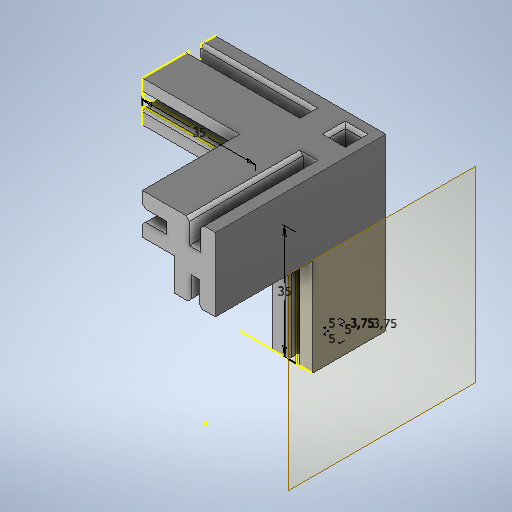
# Autodesk Inventor part: Kątownk Środek LEWY Plexa
Saved by Autodesk Inventor 2025 (Build 290162000, 162)
## iProperties
Created: 2025-07-29
Part Number: Kątownk Środek LEWY Plexa
Material: Ogólny
Document SubType Name: Modeling
Designer: ThePi
Density: 1 g/cm^3
Appearance: Domyślna
Author: ThePi
Autodesk Inventor part; units mm, degrees
(part 1 of 2)
ref_plane "YZ Plane" through (0, 0, 0) normal (1, 0, 0) x (0, 1, 0)
ref_plane "XZ Plane" through (0, 0, 0) normal (0, 1, 0) x (-1, 0, 0)
ref_plane "XY Plane" through (0, 0, 0) normal (0, 0, 1) x (1, 0, 0)
sketch "Szkic1" plane through (0, 0, 0) normal (0, 1, 0) x (-1, 0, 0)
  line L0 (0, 0) -> (0, 15)
  line L1 (0, 15) -> (0, 0)
  line L2 (0, 0) -> (15, 0)
  line L3 (3, 10) -> (4.25, 10)
  line L4 (3, 10) -> (1.75, 10)
  line L5 (1.75, 10) -> (1.75, 15)
  line L6 (4.25, 10) -> (4.25, 15)
  line L7 (1.75, 15) -> (-3.25, 15)
  line L8 (4.25, 15) -> (9.25, 15)
  line L9 (-3.25, 15) -> (-3.25, 0)
  line L10 (-3.25, 0) -> (15, 0)
  line L11 (-3.25, 0) -> (11.75, 0)
  line L12 (9.25, 15) -> (9.25, 5)
  line L13 (9.25, 5) -> (19.25, 5)
  line L14 (19.25, 5) -> (19.25, 0)
  line L15 (19.25, 0) -> (14.25, 0)
  line L16 (14.25, 0) -> (14.25, -2.5)
  line L17 (14.25, -2.5) -> (19.25, -2.5)
  line L18 (19.25, -2.5) -> (19.25, -7.5)
  line L19 (19.25, -7.5) -> (9.25, -7.5)
  line L20 (-3.25, 0) -> (-3.25, -7.5)
  line L21 (-3.25, -7.5) -> (9.25, -7.5)
  line L22 (3, 10) -> (3, -1.25)
  line L23 (3, -1.25) -> (14.25, -1.25)
  dimension "d0" = 15
  dimension "d6" = 1.25
  dimension "d7" = 1.25
  dimension "d9" = 5
  dimension "d10" = 5
  dimension "d13" = 10
  dimension "d14" = 10
  dimension "d15" = 5
  dimension "d16" = 5
  dimension "d17" = 2.5
  dimension "d18" = 5
  dimension "d19" = 10
  constraints: 48 end point, 7 perpendicular, 5 point on line, 4 vertical, 2 collinear, 2 horizontal, 1 midpoint, 1 parallel
  measures "d0" distance of L0.start L0.end
  measures "d6" distance of L3.start L3.end
  measures "d7" distance of L3.start L4.end
  measures "d9" distance of L5.end L7.end
  measures "d10" distance of L6.end L8.end
  measures "d13" distance of L8.end L12.end
  measures "d14" distance of L12.end L13.end
  measures "d15" distance of L13.end L14.end
  measures "d16" distance of L14.end L15.end
  measures "d17" distance of L15.end L16.end
  measures "d18" distance of L17.end L18.end
  measures "d19" distance of L18.end L19.end
extrude "Wyciągnięcie proste1" add sketch "Szkic1" along normal blind 30
sketch "Szkic2" plane through (0, 30, 0) normal (0, 1, 0) x (1, 0, 0)
  line L0 (3.25, 7.5) -> (-19.25, 7.5) projected
  line L1 (-19.25, -5) -> (-9.25, -5) projected
  line L2 (-19.25, 7.5) -> (-19.25, -5)
  line L3 (-19.25, -5) -> (-9.25, -5)
  line L4 (-9.25, -5) -> (-9.25, -15) projected
  line L5 (-9.25, -5) -> (-9.25, -15)
  line L6 (-1.75, -15) -> (3.25, -15) projected
  line L7 (-9.25, -15) -> (3.25, -15)
  line L8 (3.25, -15) -> (3.25, 7.5)
  line L9 (3.25, 7.5) -> (-19.25, 7.5)
  point P0 (0, 0)
  constraints: 12 end point, 3 perpendicular, 2 collinear, 1 vertical
extrude "Wyciągnięcie proste2" add sketch "Szkic2" along normal blind 30
sketch "Szkic3" plane through (0, 0, 0) normal (0, -1, 0) x (1, 0, 0)
  point P0 (0, 0)
sketch "Szkic4" plane through (-19.25, 0, -7.5) normal (-1, 0, 0) x (0, 0, 1)
  line L0 (0, 30) -> (12.5, 30)
  line L1 (12.5, 0) -> (12.5, 60) projected
  line L2 (12.5, 30) -> (12.5, 60)
  line L3 (12.5, 60) -> (0, 60)
  line L4 (0, 60) -> (0, 30)
  point P0 (7.5, 0)
  constraints: 8 end point, 2 perpendicular, 1 collinear, 1 midpoint
extrude "Wyciągnięcie proste3" add sketch "Szkic4" along normal blind 30
sketch "Szkic5" plane through (-9.25, 0, 5) normal (-1, 0, 0) x (0, 0, 1)
  line L0 (10, 0) -> (10, 60) projected
  line L1 (10, 30) -> (5, 30) projected
  line L2 (10, 60) -> (10, 30)
  line L3 (10, 30) -> (0, 30)
  line L4 (0, 30) -> (0, 60)
  line L5 (0, 60) -> (10, 60)
  point P0 (-5, 0)
  constraints: 8 end point, 2 perpendicular, 1 collinear, 1 vertical
extrude "Wyciągnięcie proste4" add sketch "Szkic5" along normal up to surface (40 mm away)
sketch "Szkic6" plane through (0, 30, 0) normal (0, -1, 0) x (1, 0, 0)
  line L0 (-14.25, 0) -> (-19.25, 0) projected
  line L1 (-14.25, 0) -> (-49.25, 0)
  line L2 (-49.25, -7.5) -> (-49.25, 15) projected
  line L3 (-49.25, 0) -> (-49.25, -2.5)
  line L4 (-49.25, -2.5) -> (-14.25, -2.5)
  line L5 (-14.25, -2.5) -> (-14.25, 0)
  line L6 (-14.25, 10) -> (-49.25, 10)
  line L7 (-4.25, 10) -> (-1.75, 10) projected
  point P0 (0, 0)
  constraints: 10 end point, 3 point on line, 2 perpendicular, 1 collinear, 1 horizontal, 1 vertical
extrude "Wyciągnięcie proste5" cut sketch "Szkic6" against normal blind 5
sketch "Szkic7" plane through (-1.75, 0, 15) normal (0, 0, 1) x (1, 0, 0)
  line L0 (-7.5, 30) -> (-17.5, 30) projected
  line L1 (-7.5, 30) -> (-17.5, 30)
  line L2 (-7.5, 30) -> (-7.5, 40)
  line L3 (5, 0) -> (5, 60) projected
  line L4 (-7.5, 30) -> (2.5, 30) construction
  line L5 (-7.5, 40) -> (-47.5, 40)
  line L6 (-47.5, 60) -> (-47.5, 30) projected
  line L7 (-47.5, 40) -> (-47.5, 30)
  line L8 (-47.5, 30) -> (-7.5, 30)
  point P0 (1.75, 0)
  dimension "d30" = 10
  dimension "d31" = 10
  dimension "d32" = 90
  constraints: 12 end point, 2 collinear, 2 perpendicular, 1 horizontal, 1 parallel, 1 point on line, 1 vertical
  measures "d30" distance of L0.start L0.end
  measures "d31" distance of L0.start L2.end
  measures "d32" angle of L4 L2
extrude "Wyciągnięcie proste6" cut sketch "Szkic7" against normal up to surface (10 mm away)
sketch "Szkic8" plane through (-49.25, 0, -7.5) normal (-1, 0, 0) x (0, 0, 1)
  point P0 (7.5, 0)
sketch "Szkic9" plane through (0, 0, 0) normal (0, -1, 0) x (1, 0, 0)
  point P0 (0, 0)
sketch "Szkic10" plane through (-49.25, 0, -7.5) normal (-1, 0, 0) x (0, 0, 1)
  line L0 (0, 0) -> (0, 60) projected
  line L1 (0, 30) -> (0, 52.5)
  line L2 (0, 52.5) -> (22.5, 52.5)
  line L3 (22.5, 0) -> (22.5, 60) projected
  line L4 (22.5, 52.5) -> (22.5, 40)
  line L5 (22.5, 40) -> (12.5, 40)
  line L6 (12.5, 40) -> (12.5, 30)
  line L7 (0, 30) -> (5, 30) projected
  line L8 (12.5, 30) -> (0, 30)
  line L9 (22.5, 52.5) -> (22.5, 60)
  line L10 (22.5, 60) -> (0, 60) projected
  line L11 (0, 60) -> (0, 52.5)
  line L12 (22.5, 52.5) -> (0, 52.5)
  point P0 (7.5, 0)
  dimension "d35" = 22.5
  dimension "d36" = 90
  dimension "d37" = 10
  constraints: 18 end point, 4 perpendicular, 3 collinear, 2 point on line, 1 midpoint
  measures "d35" distance of L1.start L1.end
  measures "d36" angle of L1 L2
  measures "d37" distance of L4.end L5.end
sketch "Szkic11" plane through (0, 0, 0) normal (0, -1, 0) x (1, 0, 0)
  point P0 (0, 0)
extrude "Wyciągnięcie proste7" cut sketch "Szkic10" against normal up to surface (52.5 mm away) contours L0 L10 L3 L2
sketch "Szkic12" plane through (-9.25, 0, 15) normal (0, 0, 1) x (1, 0, 0)
  line L0 (12.5, 52.5) -> (-40, 52.5) projected
  line L1 (12.5, 52.5) -> (-10, 52.5)
  line L2 (-10, 30) -> (-40, 30) projected
  line L3 (-10, 52.5) -> (-10, 30)
  line L4 (-10, 30) -> (12.5, 30)
  line L5 (12.5, 0) -> (12.5, 52.5) projected
  line L6 (12.5, 30) -> (12.5, 52.5)
  line L7 (-10, 30) -> (-10, 40)
  line L8 (-40, 40) -> (0, 40) projected
  line L9 (0, 40) -> (0, 30.3734)
  line L10 (0, 0) -> (0, 40) projected
  point P0 (9.25, 0)
  point P1 (0, 30)
  point P2 (0, 40)
  constraints: 12 end point, 3 perpendicular, 3 point on line, 1 parallel
extrude "Wyciągnięcie proste8" add sketch "Szkic12" against normal blind 10 contours L8 L9 L10 L4 L3
sketch "Szkic13" plane through (-9.25, 0, 15) normal (0, 0, 1) x (1, 0, 0)
  line L0 (-40, 52.5) -> (-40, 40) projected
  line L1 (-40, 40) -> (-40, 45)
  line L2 (-40, 45) -> (-10, 45)
  line L3 (-10, 45) -> (-10, 47.5)
  line L4 (-10, 47.5) -> (-40, 47.5)
  line L5 (12.5, 52.5) -> (-40, 52.5) projected
  line L6 (-40, 52.5) -> (-40, 47.5)
  line L7 (-40, 45) -> (-40, 47.5)
  point P0 (9.25, 0)
  dimension "d42" = 5
  dimension "d43" = 30
  dimension "d44" = 2.5
  constraints: 12 end point, 2 collinear, 2 perpendicular, 2 point on line, 1 horizontal
  measures "d42" distance of L0.end L1.end
  measures "d43" distance of L1.end L2.end
  measures "d44" distance of L2.end L3.end
extrude "Wyciągnięcie proste9" cut sketch "Szkic13" against normal blind 5
sketch "Szkic14" plane through (-9.25, 0, 15) normal (0, 0, 1) x (1, 0, 0)
  line L0 (12.5, 0) -> (12.5, 52.5) projected
  line L1 (12.5, 52.5) -> (-10, 52.5)
  line L2 (12.5, 52.5) -> (-40, 52.5) projected
  line L3 (-10, 40) -> (-10, 30) projected
  line L4 (-10, 52.5) -> (-10, 30)
  line L5 (-10, 30) -> (12.5, 30)
  line L6 (12.5, 30) -> (12.5, 52.5)
  point P0 (9.25, 0)
  constraints: 8 end point, 2 perpendicular, 1 point on line, 1 vertical
extrude "Wyciągnięcie proste10" add sketch "Szkic14" along normal blind 30
sketch "Szkic15" plane through (-1.75, 0, 15) normal (0, 0, 1) x (1, 0, 0)
  line L0 (0, 0) -> (0, 30) projected
  line L1 (0, 0) -> (0, 35)
  line L2 (0, 35) -> (0, 0)
  line L3 (-2.5, 0) -> (-2.5, 30) projected
  line L4 (0, 0) -> (-2.5, 0)
  line L5 (5, 0) -> (-17.5, 0) projected
  line L6 (-2.5, 0) -> (-2.5, 35)
  line L7 (-2.5, 35) -> (0, 35)
  line L8 (0, 0) -> (0, 35)
  line L9 (-17.5, 45) -> (-47.5, 45) projected
  line L10 (-47.5, 45) -> (-12.5, 45)
  line L11 (-12.5, 45) -> (-47.5, 45)
  line L12 (-47.5, 47.5) -> (-17.5, 47.5) projected
  line L13 (-47.5, 45) -> (-47.5, 47.5)
  line L14 (-47.5, 47.5) -> (-12.5, 47.5)
  line L15 (-12.5, 47.5) -> (-12.5, 45)
  point P0 (1.75, 0)
  point P1 (-17.5, 47.5)
  dimension "d49" = 35
  dimension "d50" = 35
  constraints: 22 end point, 6 collinear, 2 perpendicular, 2 vertical, 1 parallel
  measures "d49" distance of L0.start L1.end
  measures "d50" distance of L9.end L10.end
extrude "Wyciągnięcie proste11" cut sketch "Szkic15" against normal up to surface (5 mm away)
sketch "Szkic16" plane through (-9.25, 0, 45) normal (0, 0, 1) x (1, 0, 0)
  line L0 (7.5, 0) -> (7.5, 35) projected
  line L1 (7.5, 30) -> (7.5, 35)
  line L2 (5, 35) -> (5, 30) projected
  line L3 (7.5, 35) -> (5, 35)
  line L4 (5, 35) -> (5, 30)
  line L5 (5, 30) -> (7.5, 30)
  line L6 (-10, 40) -> (-10, 45) projected
  line L7 (-10, 45) -> (-5, 45) projected
  line L8 (-10, 45) -> (-5, 45)
  line L9 (-5, 47.5) -> (-10, 47.5) projected
  line L10 (-5, 45) -> (-5, 47.5)
  line L11 (-5, 47.5) -> (-10, 47.5)
  line L12 (-10, 47.5) -> (-10, 45)
  point P0 (9.25, 0)
  dimension "d53" = 5
  constraints: 16 end point, 5 perpendicular, 3 collinear, 1 point on line
  measures "d53" distance of L1.start L0.end
extrude "Wyciągnięcie proste12" cut sketch "Szkic16" against normal up to surface (35 mm away)
sketch "Szkic17" plane through (-9.25, 0, 45) normal (0, 0, 1) x (1, 0, 0)
  line L0 (-10, 30) -> (5, 30) projected
  line L1 (0, 30) -> (0, 40)
  line L2 (-40, 40) -> (-10, 40) projected
  line L3 (0, 40) -> (-10, 40)
  line L4 (-10, 40) -> (-10, 30)
  line L5 (-10, 30) -> (0, 30)
  point P0 (9.25, 0)
  dimension "d56" = 10
  constraints: 8 end point, 3 perpendicular, 1 point on line
  measures "d56" distance of L1.start L1.end
extrude "Wyciągnięcie proste13" cut sketch "Szkic17" against normal up to surface (40 mm away)
thicken "Pogrubienie1" operation cut thickness 0.5 both sides no extend neighbours no toward (-1, 0, 0) faces at (-4.25, 21.6667, 11.6667)
thicken "Pogrubienie2" operation cut thickness 0.5 both sides no extend neighbours no toward (0, 1, 0) faces at (-27.5833, 47.5, 11.6667)
thicken "Pogrubienie3" operation cut thickness 0.5 both sides no extend neighbours no toward (1, 0, 0) faces at (-1.75, 21.6667, 11.6667)
thicken "Pogrubienie4" operation cut thickness 0.5 both sides no extend neighbours no toward (0, -1, 0) faces at (-27.5833, 45, 11.6667)
thicken "Pogrubienie5" operation cut thickness 0.5 both sides no extend neighbours no toward (0, 0, -1) faces at (-15.9167, 21.6667, -2.5)
thicken "Pogrubienie6" operation cut thickness 0.5 both sides no extend neighbours no toward (0, 0, 1) faces at (-27.5833, 33.3333, 0)
sketch "Szkic21" plane through (-49.25, 0, -7.5) normal (-1, 0, 0) x (0, 0, 1)
  line L0 (4.5, 35) -> (8, 35) projected
  line L1 (4.5, 35) -> (4.5, 52.5)
  line L2 (22.5, 52.5) -> (0, 52.5) projected
  line L3 (8, 0) -> (8, 35) projected
  line L4 (8, 35) -> (8, 52.5)
  line L5 (8, 52.5) -> (4.5, 52.5)
  line L6 (4.5, 52.5) -> (4.5, 47.5)
  line L7 (4.5, 47.5) -> (8, 47.5)
  point P0 (7.5, 0)
  dimension "d92" = 5
  constraints: 10 end point, 3 point on line, 2 perpendicular, 2 vertical
  measures "d92" distance of L1.end L6.end
sketch "Szkic22" plane through (-9.25, 0, 45) normal (0, 0, 1) x (1, 0, 0)
  point P0 (9.25, 0)
sketch "Szkic23" plane through (-9.25, 0, 45) normal (0, 0, 1) x (1, 0, 0)
  line L0 (4.5, 35) -> (8, 35) projected
  line L1 (4.5, 35) -> (4.5, 52.5)
  line L2 (12.5, 52.5) -> (-10, 52.5) projected
  line L3 (8, 35) -> (8, 52.5)
  line L4 (8, 52.5) -> (4.5, 52.5)
  line L5 (4.5, 52.5) -> (4.5, 47.5)
  line L6 (4.5, 47.5) -> (8, 47.5)
  point P0 (9.25, 0)
  dimension "d93" = 5
  constraints: 10 end point, 3 point on line, 2 vertical, 1 collinear, 1 perpendicular
  measures "d93" distance of L1.end L5.end
extrude "Wyciągnięcie proste17" cut sketch "Szkic21" against normal blind 35 contours L1 L2 L4 L7
extrude "Wyciągnięcie proste18" cut sketch "Szkic23" against normal blind 35 contours L1 L2 L3 L6
sketch "Szkic25" plane through (-49.25, 52.5, -7.5) normal (0, 1, 0) x (1, 0, 0)
  line L0 (0, -8) -> (0, -4.5) projected
  line L1 (0, -4.5) -> (0, -8)
  line L2 (0, -8) -> (35, -8)
  line L3 (35, -8) -> (35, -4.5)
  line L4 (35, -4.5) -> (0, -4.5)
  point P0 (49.25, -7.5)
  constraints: 8 end point, 3 perpendicular, 1 collinear
sketch "Szkic26" plane through (-49.25, 52.5, -7.5) normal (0, 1, 0) x (1, 0, 0)
  line L0 (44.5, -17.5) -> (44.5, -22.5) projected
  line L1 (44.5, -17.5) -> (52.5, -17.5)
  line L2 (52.5, 0) -> (52.5, -52.5) projected
  line L3 (44.5, -17.5) -> (40, -17.5)
  line L4 (35, -8) -> (35, -4.5) projected
  line L5 (35, -12.5) -> (40, -12.5)
  line L6 (40, -12.5) -> (40, -17.5)
  line L7 (52.5, -22.5) -> (48, -22.5) projected
  line L8 (48, -17.5) -> (48, -22.5)
  line L9 (48, -22.5) -> (48, -12.5)
  line L10 (48, -12.5) -> (52.5, -12.5)
  line L11 (52.5, -22.5) -> (52.5, -12.5)
  line L12 (30, -8) -> (35, -8) projected
  line L13 (35, -8) -> (30, -8)
  line L14 (30, -22.5) -> (0, -22.5) projected
  line L15 (30, -22.5) -> (30, -12.5)
  line L16 (30, -12.5) -> (52.5, -12.5)
  line L17 (30, -12.5) -> (40, -12.5)
  line L18 (40, -12.5) -> (40, 0)
  line L19 (40, -52.5) -> (40, -12.5) projected
  line L20 (40, -12.5) -> (52.5, -12.5)
  line L21 (40, 0) -> (40, -12.5)
  line L22 (40, -12.5) -> (0, -12.5)
  line L23 (0, -12.5) -> (0, -8)
  line L24 (0, -8) -> (35, -8)
  line L25 (35, -8) -> (35, -4.5)
  line L26 (35, -4.5) -> (30, -4.5) projected
  line L27 (30, -4.5) -> (0, -4.5) projected
  line L28 (35, -4.5) -> (0, -4.5)
  line L29 (0, -4.5) -> (0, 0)
  line L30 (0, 0) -> (40, 0)
  line L31 (40, 0) -> (52.5, 0)
  line L32 (52.5, 0) -> (52.5, -12.5)
  line L33 (44.5, -17.5) -> (48, -17.5) projected
  line L34 (40, -12.5) -> (52.5, -12.5)
  line L35 (52.5, -52.5) -> (52.5, -12.5)
  line L36 (52.5, -52.5) -> (30, -52.5) projected
  line L37 (52.5, -52.5) -> (48, -52.5)
  line L38 (48, -17.5) -> (48, -52.5) projected
  line L39 (48, -52.5) -> (48, -17.5)
  line L40 (48, -17.5) -> (44.5, -17.5) projected
  line L41 (48, -17.5) -> (44.5, -17.5)
  line L42 (44.5, -52.5) -> (44.5, -17.5) projected
  line L43 (44.5, -17.5) -> (44.5, -52.5)
  line L44 (44.5, -52.5) -> (40, -52.5)
  line L45 (40, -52.5) -> (40, -12.5)
  point P0 (49.25, -7.5)
  dimension "d105" = 4.5
  dimension "d107" = 10
  dimension "d110" = 10
  constraints: 64 end point, 10 collinear, 9 point on line, 7 perpendicular, 3 horizontal, 1 vertical
  measures "d105" distance of L0.start L3.end
  measures "d107" distance of L7.end L9.end
  measures "d110" distance of L14.start L15.end
extrude "Wyciągnięcie proste20" [suppressed]
sketch "Szkic27" plane through (-4.75, 47.5, 45) normal (0, 1, 0) x (1, 0, 0)
  line L0 (3.5, 35) -> (0, 35)
  line L1 (-14.5, 48) -> (-44.5, 48) projected
  line L2 (-44.5, 48) -> (-44.5, 44.5) projected
  line L3 (-44.5, 48) -> (-44.5, 44.5)
  line L4 (-9.5, 48) -> (-9.5, 44.5) projected
  line L5 (-44.5, 44.5) -> (-9.5, 44.5)
  line L6 (-9.5, 44.5) -> (-9.5, 48)
  line L7 (-9.5, 48) -> (-44.5, 48.1482)
  line L8 (3.5, 0) -> (3.5, 35) projected
  line L9 (3.5, 0) -> (0, 0) projected
  line L10 (3.5, 0) -> (0, 0)
  line L11 (0, 0) -> (0, 35)
  line L12 (0, 35) -> (3.5, 35)
  line L13 (3.5, 0) -> (3.5, 35)
  point P0 (4.75, 45)
  constraints: 18 end point, 4 perpendicular, 3 collinear, 1 point on line
extrude "Wyciągnięcie proste21" [suppressed]
extrude "Wyciągnięcie proste22" [suppressed]
sketch "Szkic29" plane through (-49.25, 62.5, -7.5) normal (0, 1, 0) x (1, 0, 0)
  line L0 (52.5, 0) -> (0, 0) projected
  line L1 (52.5, 0) -> (48.75, 0)
  line L2 (48.75, 0) -> (52.5, 0)
  line L3 (52.5, 0) -> (48.75, 0)
  line L4 (48.75, -3.75) -> (43.75, -3.75)
  line L5 (43.75, -3.75) -> (43.75, -8.75)
  line L6 (43.75, -8.75) -> (48.75, -8.75)
  line L7 (48.75, -8.75) -> (48.75, -3.75)
  point P0 (49.25, -7.5)
  dimension "d124" = 5
  constraints: 14 end point, 2 collinear, 1 perpendicular, 1 point on line
  measures "d124" distance of L4.start L4.end
extrude "Wyciągnięcie proste24" [suppressed]
sketch "Szkic30" plane through (0, 0, 0) normal (0, -1, 0) x (1, 0, 0)
  line L0 (3.25, -7.5) -> (-49.25, -7.5) projected
  line L1 (3.25, -7.5) -> (-0.5, -7.5)
  line L2 (-0.5, -7.5) -> (-0.5, -3.75)
  line L3 (-0.5, 1.25) -> (-5.5, 1.25) projected
  line L4 (-0.5, 1.25) -> (-0.5, -3.75)
  line L5 (-5.5, 1.25) -> (-5.5, -3.75) projected
  line L6 (-5.5, 1.2502) -> (-5.5, -3.75)
  line L7 (-5.5, -3.75) -> (-0.5, -3.75)
  point P0 (0, 0)
  dimension "d129" = 3.75
  dimension "d130" = 3.75
  constraints: 10 end point, 1 collinear, 1 perpendicular, 1 point on line
  measures "d129" distance of L0.start L1.end
  measures "d130" distance of L1.end L2.end
extrude "Wyciągnięcie proste25" [suppressed]
sketch "Szkic31" plane through (-49.25, 52.5, -7.5) normal (0, 1, 0) x (1, 0, 0)
  line L0 (0, 0) -> (52.5, 0) projected
  line L1 (52.5, 0) -> (48.75, 0)
  line L2 (48.75, 0) -> (48.75, -3.75)
  line L3 (52.5, 0) -> (48.75, 0)
  line L4 (48.75, 0) -> (48.75, -3.75)
  line L5 (48.75, -3.75) -> (43.75, -3.75)
  line L6 (43.75, -3.75) -> (43.75, -8.75)
  line L7 (43.75, -8.75) -> (48.75, -8.75)
  line L8 (48.75, -8.75) -> (48.75, -3.75)
  point P0 (49.25, -7.5)
  dimension "d135" = 3.75
  dimension "d136" = 3.75
  dimension "d137" = 5
  dimension "d138" = 5
  dimension "d139" = 5
  constraints: 16 end point, 3 perpendicular, 2 collinear, 2 point on line
  measures "d135" distance of L0.end L1.end
  measures "d136" distance of L1.end L2.end
  measures "d137" distance of L2.end L5.end
  measures "d138" distance of L5.end L6.end
  measures "d139" distance of L6.end L7.end
extrude "Wyciągnięcie proste26" cut sketch "Szkic31" against normal blind 17
sketch "Szkic32" plane through (0, 0, 0) normal (0, -1, 0) x (1, 0, 0)
  line L0 (-49.25, -7.5) -> (3.25, -7.5) projected
  line L1 (3.25, -7.5) -> (-0.5, -7.5)
  line L2 (-0.5, -7.5) -> (-4.25, -7.5)
  line L3 (-4.25, -7.5) -> (-0.5, -7.5)
  line L4 (-0.5, -7.5) -> (-0.5, -3.75)
  line L5 (-0.5, -3.75) -> (-5.5, -3.75)
  line L6 (-5.5, -3.75) -> (-5.5, 1.25)
  line L7 (-5.5, 1.25) -> (-0.5, 1.25)
  line L8 (-0.5, 1.25) -> (-0.5, -3.75)
  point P0 (0, 0)
  dimension "d142" = 3.75
  dimension "d143" = 3.75
  dimension "d144" = 3.75
  dimension "d145" = 5
  dimension "d146" = 5
  dimension "d147" = 5
  constraints: 16 end point, 3 perpendicular, 3 point on line, 2 collinear
  measures "d142" distance of L0.end L1.end
  measures "d143" distance of L1.end L2.end
  measures "d144" distance of L1.end L4.end
  measures "d145" distance of L4.end L5.end
  measures "d146" distance of L5.end L6.end
  measures "d147" distance of L6.end L7.end
extrude "Wyciągnięcie proste27" cut sketch "Szkic32" against normal blind 17
sketch "Szkic33" plane through (-49.25, 0, -7.5) normal (-1, 0, 0) x (0, 0, 1)
  line L0 (4.5, 30) -> (4.5, 35) projected
  line L1 (4.5, 35) -> (8, 35) projected
  line L2 (8, 35) -> (8, 30) projected
  line L3 (8, 30) -> (12.5, 30) projected
  line L4 (12.5, 30) -> (12.5, 40) projected
  line L5 (12.5, 40) -> (22.5, 40) projected
  line L6 (22.5, 44.5) -> (22.5, 40) projected
  line L7 (22.5, 44.5) -> (17.5, 44.5) projected
  line L8 (17.5, 44.5) -> (17.5, 48) projected
  line L9 (17.5, 48) -> (22.5, 48) projected
  line L10 (22.5, 52.5) -> (22.5, 48) projected
  line L11 (4.5, 52.5) -> (0, 52.5) projected
  line L12 (8, 52.5) -> (8, 47.5) projected
  line L13 (8, 47.5) -> (4.5, 47.5) projected
  line L14 (4.5, 47.5) -> (4.5, 52.5) projected
  line L15 (22.5, 52.5) -> (8, 52.5) projected
  line L16 (0, 52.5) -> (0, 30) projected
  line L17 (0, 30) -> (4.5, 30) projected
  point P0 (7.5, 0)
thicken "Pogrubienie8" operation cut thickness 2.5 both sides no extend neighbours no toward (0, 0, -1) faces at (-3.5833, 23.3333, 10) (-3.5833, 35, 21.6667)
thicken "Pogrubienie9" operation cut thickness 2.5 both sides no extend neighbours no toward (1, 0, 0) faces at (-14.25, 11.6667, -0.6667) (-25.9167, 35, -0.6667)
thicken "Pogrubienie10" operation cut thickness 2.5 both sides no extend neighbours no toward (0, -1, 0) faces at (-37.5833, 47.5, -1.8333)
thicken "Pogrubienie11" operation cut thickness 2.5 both sides no extend neighbours no toward (1, 0, 0) faces at (-14.25, 45.6667, 21.6667) (-25.9167, 46.8333, 10)
chamfer "Faza6" distance 1 angle 45 8 edges at (-3, 0, 1.25) (-0.5, 0, -1.25) (-3, 0, -3.75) (-5.5, 0, -1.25) (-5.5, 52.5, -1.25) (-3, 52.5, -3.75) (-0.5, 52.5, -1.25) (-3, 52.5, 1.25)
thicken "Pogrubienie12" operation cut thickness 2.5 both sides no extend neighbours no toward (0, -1, 0) faces at (-3.5833, 47.5, 33.3333)
chamfer "Faza7" distance 1 angle 45 4 edges at (-19.25, 48, 30) (-19.25, 44.5, 30) (-34.25, 48, 15) (-34.25, 44.5, 15)
chamfer "Faza13" distance 1 angle 45 6 edges at (-34.25, 30, -3) (-34.25, 30, 0.5) (-19.25, 15, -3) (-19.25, 15, 0.5) (-31.75, 52.5, -3) (-31.75, 52.5, 0.5)
thicken "Pogrubienie17" operation add thickness 0.5 both sides no extend neighbours no toward (1, 0, 0) faces at (-4.75, 35, 22.5)
thicken "Pogrubienie18" operation add thickness 0.5 both sides no extend neighbours no toward (-1, 0, 0) faces at (-1.25, 22.5, 10)
chamfer "Faza14" distance 1 angle 45 4 edges at (-4.25, 15, 15) (-1.75, 15, 15) (-1.75, 30, 30) (-4.25, 30, 30)
chamfer "Faza15" distance 1 angle 45 2 edges at (-1.25, 52.5, 27.5) (-4.75, 52.5, 27.5)
ref_plane "Płaszczyzna konstrukcyjna1" through (28.25, 0, 15) normal (1, 0, 0) x (0, 0, -1)
sketch "Szkic34" plane through (3.25, 0, 15) normal (1, 0, 0) x (0, 0, -1)
  line L0 (-5.75, 29.567) -> (-3.25, 33.8971)
  line L1 (-3.25, 33.8971) -> (1.75, 33.8971)
  line L2 (1.75, 33.8971) -> (4.25, 29.567)
  line L3 (4.25, 29.567) -> (1.75, 25.2369)
  line L4 (1.75, 25.2369) -> (-3.25, 25.2369)
  line L5 (-3.25, 25.2369) -> (-5.75, 29.567)
  line L6 (-11.25, 20.0407) -> (-8.75, 24.3708)
  line L7 (-8.75, 24.3708) -> (-3.75, 24.3708)
  line L8 (-3.75, 24.3708) -> (-1.25, 20.0407)
  line L9 (-1.25, 20.0407) -> (-3.75, 15.7106)
  line L10 (-3.75, 15.7106) -> (-8.75, 15.7106)
  line L11 (-8.75, 15.7106) -> (-11.25, 20.0407)
  line L12 (-0.25, 39.0933) -> (2.25, 43.4234)
  line L13 (2.25, 43.4234) -> (7.25, 43.4234)
  line L14 (7.25, 43.4234) -> (9.75, 39.0933)
  line L15 (9.75, 39.0933) -> (7.25, 34.7631)
  line L16 (7.25, 34.7631) -> (2.25, 34.7631)
  line L17 (2.25, 34.7631) -> (-0.25, 39.0933)
  line L18 (-16.75, 10.5144) -> (-14.25, 14.8446)
  line L19 (-14.25, 14.8446) -> (-9.25, 14.8446)
  line L20 (-9.25, 14.8446) -> (-6.75, 10.5144)
  line L21 (-6.75, 10.5144) -> (-9.25, 6.1843)
  line L22 (-9.25, 6.1843) -> (-14.25, 6.1843)
  line L23 (-14.25, 6.1843) -> (-16.75, 10.5144)
  line L24 (5.25, 48.6195) -> (7.75, 52.9497)
  line L25 (7.75, 52.9497) -> (12.75, 52.9497)
  line L26 (12.75, 52.9497) -> (15.25, 48.6195)
  line L27 (15.25, 48.6195) -> (12.75, 44.2894)
  line L28 (12.75, 44.2894) -> (7.75, 44.2894)
  line L29 (7.75, 44.2894) -> (5.25, 48.6195)
  line L30 (-22.25, 0.9881) -> (-19.75, 5.3183)
  line L31 (-19.75, 5.3183) -> (-14.75, 5.3183)
  line L32 (-14.75, 5.3183) -> (-12.25, 0.9881)
  line L33 (-12.25, 0.9881) -> (-14.75, -3.342)
  line L34 (-14.75, -3.342) -> (-19.75, -3.342)
  line L35 (-19.75, -3.342) -> (-22.25, 0.9881)
  line L36 (10.75, 58.1458) -> (13.25, 62.476)
  line L37 (13.25, 62.476) -> (18.25, 62.476)
  line L38 (18.25, 62.476) -> (20.75, 58.1458)
  line L39 (20.75, 58.1458) -> (18.25, 53.8157)
  line L40 (18.25, 53.8157) -> (13.25, 53.8157)
  line L41 (13.25, 53.8157) -> (10.75, 58.1458)
  line L42 (-27.75, -8.5381) -> (-25.25, -4.208)
  line L43 (-25.25, -4.208) -> (-20.25, -4.208)
  line L44 (-20.25, -4.208) -> (-17.75, -8.5381)
  line L45 (-17.75, -8.5381) -> (-20.25, -12.8683)
  line L46 (-20.25, -12.8683) -> (-25.25, -12.8683)
  line L47 (-25.25, -12.8683) -> (-27.75, -8.5381)
  line L48 (16.25, 67.6721) -> (18.75, 72.0022)
  line L49 (18.75, 72.0022) -> (23.75, 72.0022)
  line L50 (23.75, 72.0022) -> (26.25, 67.6721)
  line L51 (26.25, 67.6721) -> (23.75, 63.342)
  line L52 (23.75, 63.342) -> (18.75, 63.342)
  line L53 (18.75, 63.342) -> (16.25, 67.6721)
  line L54 (-33.25, -18.0644) -> (-30.75, -13.7343)
  line L55 (-30.75, -13.7343) -> (-25.75, -13.7343)
  line L56 (-25.75, -13.7343) -> (-23.25, -18.0644)
  line L57 (-23.25, -18.0644) -> (-25.75, -22.3945)
  line L58 (-25.75, -22.3945) -> (-30.75, -22.3945)
  line L59 (-30.75, -22.3945) -> (-33.25, -18.0644)
  line L60 (-0.25, 20.0407) -> (2.25, 24.3708)
  line L61 (2.25, 24.3708) -> (7.25, 24.3708)
  line L62 (7.25, 24.3708) -> (9.75, 20.0407)
  line L63 (9.75, 20.0407) -> (7.25, 15.7106)
  line L64 (7.25, 15.7106) -> (2.25, 15.7106)
  line L65 (2.25, 15.7106) -> (-0.25, 20.0407)
  line L66 (-5.75, 10.5144) -> (-3.25, 14.8446)
  line L67 (-3.25, 14.8446) -> (1.75, 14.8446)
  line L68 (1.75, 14.8446) -> (4.25, 10.5144)
  line L69 (4.25, 10.5144) -> (1.75, 6.1843)
  line L70 (1.75, 6.1843) -> (-3.25, 6.1843)
  line L71 (-3.25, 6.1843) -> (-5.75, 10.5144)
  line L72 (5.25, 29.567) -> (7.75, 33.8971)
  line L73 (7.75, 33.8971) -> (12.75, 33.8971)
  line L74 (12.75, 33.8971) -> (15.25, 29.567)
  line L75 (15.25, 29.567) -> (12.75, 25.2369)
  line L76 (12.75, 25.2369) -> (7.75, 25.2369)
  line L77 (7.75, 25.2369) -> (5.25, 29.567)
  line L78 (-11.25, 0.9881) -> (-8.75, 5.3183)
  line L79 (-8.75, 5.3183) -> (-3.75, 5.3183)
  line L80 (-3.75, 5.3183) -> (-1.25, 0.9881)
  line L81 (-1.25, 0.9881) -> (-3.75, -3.342)
  line L82 (-3.75, -3.342) -> (-8.75, -3.342)
  line L83 (-8.75, -3.342) -> (-11.25, 0.9881)
  line L84 (10.75, 39.0933) -> (13.25, 43.4234)
  line L85 (13.25, 43.4234) -> (18.25, 43.4234)
  line L86 (18.25, 43.4234) -> (20.75, 39.0933)
  line L87 (20.75, 39.0933) -> (18.25, 34.7631)
  line L88 (18.25, 34.7631) -> (13.25, 34.7631)
  line L89 (13.25, 34.7631) -> (10.75, 39.0933)
  line L90 (-16.75, -8.5381) -> (-14.25, -4.208)
  line L91 (-14.25, -4.208) -> (-9.25, -4.208)
  line L92 (-9.25, -4.208) -> (-6.75, -8.5381)
  line L93 (-6.75, -8.5381) -> (-9.25, -12.8683)
  line L94 (-9.25, -12.8683) -> (-14.25, -12.8683)
  line L95 (-14.25, -12.8683) -> (-16.75, -8.5381)
  line L96 (16.25, 48.6195) -> (18.75, 52.9497)
  line L97 (18.75, 52.9497) -> (23.75, 52.9497)
  line L98 (23.75, 52.9497) -> (26.25, 48.6195)
  line L99 (26.25, 48.6195) -> (23.75, 44.2894)
  line L100 (23.75, 44.2894) -> (18.75, 44.2894)
  line L101 (18.75, 44.2894) -> (16.25, 48.6195)
  line L102 (-22.25, -18.0644) -> (-19.75, -13.7343)
  line L103 (-19.75, -13.7343) -> (-14.75, -13.7343)
  line L104 (-14.75, -13.7343) -> (-12.25, -18.0644)
  line L105 (-12.25, -18.0644) -> (-14.75, -22.3945)
  line L106 (-14.75, -22.3945) -> (-19.75, -22.3945)
  line L107 (-19.75, -22.3945) -> (-22.25, -18.0644)
  line L108 (21.75, 58.1458) -> (24.25, 62.476)
  line L109 (24.25, 62.476) -> (29.25, 62.476)
  line L110 (29.25, 62.476) -> (31.75, 58.1458)
  line L111 (31.75, 58.1458) -> (29.25, 53.8157)
  line L112 (29.25, 53.8157) -> (24.25, 53.8157)
  line L113 (24.25, 53.8157) -> (21.75, 58.1458)
  line L114 (-27.75, -27.5907) -> (-25.25, -23.2606)
  line L115 (-25.25, -23.2606) -> (-20.25, -23.2606)
  line L116 (-20.25, -23.2606) -> (-17.75, -27.5907)
  line L117 (-17.75, -27.5907) -> (-20.25, -31.9208)
  line L118 (-20.25, -31.9208) -> (-25.25, -31.9208)
  line L119 (-25.25, -31.9208) -> (-27.75, -27.5907)
  line L120 (-11.25, 39.0933) -> (-8.75, 43.4234)
  line L121 (-8.75, 43.4234) -> (-3.75, 43.4234)
  line L122 (-3.75, 43.4234) -> (-1.25, 39.0933)
  line L123 (-1.25, 39.0933) -> (-3.75, 34.7631)
  line L124 (-3.75, 34.7631) -> (-8.75, 34.7631)
  line L125 (-8.75, 34.7631) -> (-11.25, 39.0933)
  line L126 (-16.75, 29.567) -> (-14.25, 33.8971)
  line L127 (-14.25, 33.8971) -> (-9.25, 33.8971)
  line L128 (-9.25, 33.8971) -> (-6.75, 29.567)
  line L129 (-6.75, 29.567) -> (-9.25, 25.2369)
  line L130 (-9.25, 25.2369) -> (-14.25, 25.2369)
  line L131 (-14.25, 25.2369) -> (-16.75, 29.567)
  line L132 (-5.75, 48.6195) -> (-3.25, 52.9497)
  line L133 (-3.25, 52.9497) -> (1.75, 52.9497)
  line L134 (1.75, 52.9497) -> (4.25, 48.6195)
  line L135 (4.25, 48.6195) -> (1.75, 44.2894)
  line L136 (1.75, 44.2894) -> (-3.25, 44.2894)
  line L137 (-3.25, 44.2894) -> (-5.75, 48.6195)
  line L138 (-22.25, 20.0407) -> (-19.75, 24.3708)
  line L139 (-19.75, 24.3708) -> (-14.75, 24.3708)
  line L140 (-14.75, 24.3708) -> (-12.25, 20.0407)
  line L141 (-12.25, 20.0407) -> (-14.75, 15.7106)
  line L142 (-14.75, 15.7106) -> (-19.75, 15.7106)
  line L143 (-19.75, 15.7106) -> (-22.25, 20.0407)
  line L144 (-0.25, 58.1458) -> (2.25, 62.476)
  line L145 (2.25, 62.476) -> (7.25, 62.476)
  line L146 (7.25, 62.476) -> (9.75, 58.1458)
  line L147 (9.75, 58.1458) -> (7.25, 53.8157)
  line L148 (7.25, 53.8157) -> (2.25, 53.8157)
  line L149 (2.25, 53.8157) -> (-0.25, 58.1458)
  line L150 (-27.75, 10.5144) -> (-25.25, 14.8446)
  line L151 (-25.25, 14.8446) -> (-20.25, 14.8446)
  line L152 (-20.25, 14.8446) -> (-17.75, 10.5144)
  line L153 (-17.75, 10.5144) -> (-20.25, 6.1843)
  line L154 (-20.25, 6.1843) -> (-25.25, 6.1843)
  line L155 (-25.25, 6.1843) -> (-27.75, 10.5144)
  line L156 (5.25, 67.6721) -> (7.75, 72.0022)
  line L157 (7.75, 72.0022) -> (12.75, 72.0022)
  line L158 (12.75, 72.0022) -> (15.25, 67.6721)
  line L159 (15.25, 67.6721) -> (12.75, 63.342)
  line L160 (12.75, 63.342) -> (7.75, 63.342)
  line L161 (7.75, 63.342) -> (5.25, 67.6721)
  line L162 (-33.25, 0.9881) -> (-30.75, 5.3183)
  line L163 (-30.75, 5.3183) -> (-25.75, 5.3183)
  line L164 (-25.75, 5.3183) -> (-23.25, 0.9881)
  line L165 (-23.25, 0.9881) -> (-25.75, -3.342)
  line L166 (-25.75, -3.342) -> (-30.75, -3.342)
  line L167 (-30.75, -3.342) -> (-33.25, 0.9881)
  line L168 (10.75, 77.1984) -> (13.25, 81.5285)
  line L169 (13.25, 81.5285) -> (18.25, 81.5285)
  line L170 (18.25, 81.5285) -> (20.75, 77.1984)
  line L171 (20.75, 77.1984) -> (18.25, 72.8683)
  line L172 (18.25, 72.8683) -> (13.25, 72.8683)
  line L173 (13.25, 72.8683) -> (10.75, 77.1984)
  line L174 (-38.75, -8.5381) -> (-36.25, -4.208)
  line L175 (-36.25, -4.208) -> (-31.25, -4.208)
  line L176 (-31.25, -4.208) -> (-28.75, -8.5381)
  line L177 (-28.75, -8.5381) -> (-31.25, -12.8683)
  line L178 (-31.25, -12.8683) -> (-36.25, -12.8683)
  line L179 (-36.25, -12.8683) -> (-38.75, -8.5381)
  line L180 (5.25, 10.5144) -> (7.75, 14.8446)
  line L181 (7.75, 14.8446) -> (12.75, 14.8446)
  line L182 (12.75, 14.8446) -> (15.25, 10.5144)
  line L183 (15.25, 10.5144) -> (12.75, 6.1843)
  line L184 (12.75, 6.1843) -> (7.75, 6.1843)
  line L185 (7.75, 6.1843) -> (5.25, 10.5144)
  line L186 (-0.25, 0.9881) -> (2.25, 5.3183)
  line L187 (2.25, 5.3183) -> (7.25, 5.3183)
  line L188 (7.25, 5.3183) -> (9.75, 0.9881)
  line L189 (9.75, 0.9881) -> (7.25, -3.342)
  line L190 (7.25, -3.342) -> (2.25, -3.342)
  line L191 (2.25, -3.342) -> (-0.25, 0.9881)
  line L192 (10.75, 20.0407) -> (13.25, 24.3708)
  line L193 (13.25, 24.3708) -> (18.25, 24.3708)
  line L194 (18.25, 24.3708) -> (20.75, 20.0407)
  line L195 (20.75, 20.0407) -> (18.25, 15.7106)
  line L196 (18.25, 15.7106) -> (13.25, 15.7106)
  line L197 (13.25, 15.7106) -> (10.75, 20.0407)
  line L198 (-5.75, -8.5381) -> (-3.25, -4.208)
  line L199 (-3.25, -4.208) -> (1.75, -4.208)
  line L200 (1.75, -4.208) -> (4.25, -8.5381)
  line L201 (4.25, -8.5381) -> (1.75, -12.8683)
  line L202 (1.75, -12.8683) -> (-3.25, -12.8683)
  line L203 (-3.25, -12.8683) -> (-5.75, -8.5381)
  line L204 (16.25, 29.567) -> (18.75, 33.8971)
  line L205 (18.75, 33.8971) -> (23.75, 33.8971)
  line L206 (23.75, 33.8971) -> (26.25, 29.567)
  line L207 (26.25, 29.567) -> (23.75, 25.2369)
  line L208 (23.75, 25.2369) -> (18.75, 25.2369)
  line L209 (18.75, 25.2369) -> (16.25, 29.567)
  line L210 (-11.25, -18.0644) -> (-8.75, -13.7343)
  line L211 (-8.75, -13.7343) -> (-3.75, -13.7343)
  line L212 (-3.75, -13.7343) -> (-1.25, -18.0644)
  line L213 (-1.25, -18.0644) -> (-3.75, -22.3945)
  line L214 (-3.75, -22.3945) -> (-8.75, -22.3945)
  line L215 (-8.75, -22.3945) -> (-11.25, -18.0644)
  line L216 (21.75, 39.0933) -> (24.25, 43.4234)
  line L217 (24.25, 43.4234) -> (29.25, 43.4234)
  line L218 (29.25, 43.4234) -> (31.75, 39.0933)
  line L219 (31.75, 39.0933) -> (29.25, 34.7631)
  line L220 (29.25, 34.7631) -> (24.25, 34.7631)
  line L221 (24.25, 34.7631) -> (21.75, 39.0933)
  line L222 (-16.75, -27.5907) -> (-14.25, -23.2606)
  line L223 (-14.25, -23.2606) -> (-9.25, -23.2606)
  line L224 (-9.25, -23.2606) -> (-6.75, -27.5907)
  line L225 (-6.75, -27.5907) -> (-9.25, -31.9208)
  line L226 (-9.25, -31.9208) -> (-14.25, -31.9208)
  line L227 (-14.25, -31.9208) -> (-16.75, -27.5907)
  line L228 (27.25, 48.6195) -> (29.75, 52.9497)
  line L229 (29.75, 52.9497) -> (34.75, 52.9497)
  line L230 (34.75, 52.9497) -> (37.25, 48.6195)
  line L231 (37.25, 48.6195) -> (34.75, 44.2894)
  line L232 (34.75, 44.2894) -> (29.75, 44.2894)
  line L233 (29.75, 44.2894) -> (27.25, 48.6195)
  line L234 (-22.25, -37.117) -> (-19.75, -32.7868)
  line L235 (-19.75, -32.7868) -> (-14.75, -32.7868)
  line L236 (-14.75, -32.7868) -> (-12.25, -37.117)
  line L237 (-12.25, -37.117) -> (-14.75, -41.4471)
  line L238 (-14.75, -41.4471) -> (-19.75, -41.4471)
  line L239 (-19.75, -41.4471) -> (-22.25, -37.117)
  line L240 (-16.75, 48.6195) -> (-14.25, 52.9497)
  line L241 (-14.25, 52.9497) -> (-9.25, 52.9497)
  line L242 (-9.25, 52.9497) -> (-6.75, 48.6195)
  line L243 (-6.75, 48.6195) -> (-9.25, 44.2894)
  line L244 (-9.25, 44.2894) -> (-14.25, 44.2894)
  line L245 (-14.25, 44.2894) -> (-16.75, 48.6195)
  line L246 (-22.25, 39.0933) -> (-19.75, 43.4234)
  line L247 (-19.75, 43.4234) -> (-14.75, 43.4234)
  line L248 (-14.75, 43.4234) -> (-12.25, 39.0933)
  line L249 (-12.25, 39.0933) -> (-14.75, 34.7631)
  line L250 (-14.75, 34.7631) -> (-19.75, 34.7631)
  line L251 (-19.75, 34.7631) -> (-22.25, 39.0933)
  line L252 (-11.25, 58.1458) -> (-8.75, 62.476)
  line L253 (-8.75, 62.476) -> (-3.75, 62.476)
  line L254 (-3.75, 62.476) -> (-1.25, 58.1458)
  line L255 (-1.25, 58.1458) -> (-3.75, 53.8157)
  line L256 (-3.75, 53.8157) -> (-8.75, 53.8157)
  line L257 (-8.75, 53.8157) -> (-11.25, 58.1458)
  line L258 (-27.75, 29.567) -> (-25.25, 33.8971)
  line L259 (-25.25, 33.8971) -> (-20.25, 33.8971)
  line L260 (-20.25, 33.8971) -> (-17.75, 29.567)
  line L261 (-17.75, 29.567) -> (-20.25, 25.2369)
  line L262 (-20.25, 25.2369) -> (-25.25, 25.2369)
  line L263 (-25.25, 25.2369) -> (-27.75, 29.567)
  line L264 (-5.75, 67.6721) -> (-3.25, 72.0022)
  line L265 (-3.25, 72.0022) -> (1.75, 72.0022)
  line L266 (1.75, 72.0022) -> (4.25, 67.6721)
  line L267 (4.25, 67.6721) -> (1.75, 63.342)
  line L268 (1.75, 63.342) -> (-3.25, 63.342)
  line L269 (-3.25, 63.342) -> (-5.75, 67.6721)
  line L270 (-33.25, 20.0407) -> (-30.75, 24.3708)
  line L271 (-30.75, 24.3708) -> (-25.75, 24.3708)
  line L272 (-25.75, 24.3708) -> (-23.25, 20.0407)
  line L273 (-23.25, 20.0407) -> (-25.75, 15.7106)
  line L274 (-25.75, 15.7106) -> (-30.75, 15.7106)
  line L275 (-30.75, 15.7106) -> (-33.25, 20.0407)
  line L276 (-0.25, 77.1984) -> (2.25, 81.5285)
  line L277 (2.25, 81.5285) -> (7.25, 81.5285)
  line L278 (7.25, 81.5285) -> (9.75, 77.1984)
  line L279 (9.75, 77.1984) -> (7.25, 72.8683)
  line L280 (7.25, 72.8683) -> (2.25, 72.8683)
  line L281 (2.25, 72.8683) -> (-0.25, 77.1984)
  line L282 (-38.75, 10.5144) -> (-36.25, 14.8446)
  line L283 (-36.25, 14.8446) -> (-31.25, 14.8446)
  line L284 (-31.25, 14.8446) -> (-28.75, 10.5144)
  line L285 (-28.75, 10.5144) -> (-31.25, 6.1843)
  line L286 (-31.25, 6.1843) -> (-36.25, 6.1843)
  line L287 (-36.25, 6.1843) -> (-38.75, 10.5144)
  line L288 (5.25, 86.7247) -> (7.75, 91.0548)
  line L289 (7.75, 91.0548) -> (12.75, 91.0548)
  line L290 (12.75, 91.0548) -> (15.25, 86.7247)
  line L291 (15.25, 86.7247) -> (12.75, 82.3945)
  line L292 (12.75, 82.3945) -> (7.75, 82.3945)
  line L293 (7.75, 82.3945) -> (5.25, 86.7247)
  line L294 (-44.25, 0.9881) -> (-41.75, 5.3183)
  line L295 (-41.75, 5.3183) -> (-36.75, 5.3183)
  line L296 (-36.75, 5.3183) -> (-34.25, 0.9881)
  line L297 (-34.25, 0.9881) -> (-36.75, -3.342)
  line L298 (-36.75, -3.342) -> (-41.75, -3.342)
  line L299 (-41.75, -3.342) -> (-44.25, 0.9881)
  line L300 (10.75, 0.9881) -> (13.25, 5.3183)
  line L301 (13.25, 5.3183) -> (18.25, 5.3183)
  line L302 (18.25, 5.3183) -> (20.75, 0.9881)
  line L303 (20.75, 0.9881) -> (18.25, -3.342)
  line L304 (18.25, -3.342) -> (13.25, -3.342)
  line L305 (13.25, -3.342) -> (10.75, 0.9881)
  line L306 (5.25, -8.5381) -> (7.75, -4.208)
  line L307 (7.75, -4.208) -> (12.75, -4.208)
  line L308 (12.75, -4.208) -> (15.25, -8.5381)
  line L309 (15.25, -8.5381) -> (12.75, -12.8683)
  line L310 (12.75, -12.8683) -> (7.75, -12.8683)
  line L311 (7.75, -12.8683) -> (5.25, -8.5381)
  line L312 (16.25, 10.5144) -> (18.75, 14.8446)
  line L313 (18.75, 14.8446) -> (23.75, 14.8446)
  line L314 (23.75, 14.8446) -> (26.25, 10.5144)
  line L315 (26.25, 10.5144) -> (23.75, 6.1843)
  line L316 (23.75, 6.1843) -> (18.75, 6.1843)
  line L317 (18.75, 6.1843) -> (16.25, 10.5144)
  line L318 (-0.25, -18.0644) -> (2.25, -13.7343)
  line L319 (2.25, -13.7343) -> (7.25, -13.7343)
  line L320 (7.25, -13.7343) -> (9.75, -18.0644)
  line L321 (9.75, -18.0644) -> (7.25, -22.3945)
  line L322 (7.25, -22.3945) -> (2.25, -22.3945)
  line L323 (2.25, -22.3945) -> (-0.25, -18.0644)
  line L324 (21.75, 20.0407) -> (24.25, 24.3708)
  line L325 (24.25, 24.3708) -> (29.25, 24.3708)
  line L326 (29.25, 24.3708) -> (31.75, 20.0407)
  line L327 (31.75, 20.0407) -> (29.25, 15.7106)
  line L328 (29.25, 15.7106) -> (24.25, 15.7106)
  line L329 (24.25, 15.7106) -> (21.75, 20.0407)
  line L330 (-5.75, -27.5907) -> (-3.25, -23.2606)
  line L331 (-3.25, -23.2606) -> (1.75, -23.2606)
  line L332 (1.75, -23.2606) -> (4.25, -27.5907)
  line L333 (4.25, -27.5907) -> (1.75, -31.9208)
  line L334 (1.75, -31.9208) -> (-3.25, -31.9208)
  line L335 (-3.25, -31.9208) -> (-5.75, -27.5907)
  line L336 (27.25, 29.567) -> (29.75, 33.8971)
  line L337 (29.75, 33.8971) -> (34.75, 33.8971)
  line L338 (34.75, 33.8971) -> (37.25, 29.567)
  line L339 (37.25, 29.567) -> (34.75, 25.2369)
  line L340 (34.75, 25.2369) -> (29.75, 25.2369)
  line L341 (29.75, 25.2369) -> (27.25, 29.567)
  line L342 (-11.25, -37.117) -> (-8.75, -32.7868)
  line L343 (-8.75, -32.7868) -> (-3.75, -32.7868)
  line L344 (-3.75, -32.7868) -> (-1.25, -37.117)
  line L345 (-1.25, -37.117) -> (-3.75, -41.4471)
  line L346 (-3.75, -41.4471) -> (-8.75, -41.4471)
  line L347 (-8.75, -41.4471) -> (-11.25, -37.117)
  line L348 (32.75, 39.0933) -> (35.25, 43.4234)
  line L349 (35.25, 43.4234) -> (40.25, 43.4234)
  line L350 (40.25, 43.4234) -> (42.75, 39.0933)
  line L351 (42.75, 39.0933) -> (40.25, 34.7631)
  line L352 (40.25, 34.7631) -> (35.25, 34.7631)
  line L353 (35.25, 34.7631) -> (32.75, 39.0933)
  line L354 (-16.75, -46.6432) -> (-14.25, -42.3131)
  line L355 (-14.25, -42.3131) -> (-9.25, -42.3131)
  line L356 (-9.25, -42.3131) -> (-6.75, -46.6432)
  line L357 (-6.75, -46.6432) -> (-9.25, -50.9734)
  line L358 (-9.25, -50.9734) -> (-14.25, -50.9734)
  line L359 (-14.25, -50.9734) -> (-16.75, -46.6432)
  line L360 (-22.25, 58.1458) -> (-19.75, 62.476)
  line L361 (-19.75, 62.476) -> (-14.75, 62.476)
  line L362 (-14.75, 62.476) -> (-12.25, 58.1458)
  line L363 (-12.25, 58.1458) -> (-14.75, 53.8157)
  line L364 (-14.75, 53.8157) -> (-19.75, 53.8157)
  line L365 (-19.75, 53.8157) -> (-22.25, 58.1458)
  line L366 (-27.75, 48.6195) -> (-25.25, 52.9497)
  line L367 (-25.25, 52.9497) -> (-20.25, 52.9497)
  line L368 (-20.25, 52.9497) -> (-17.75, 48.6195)
  line L369 (-17.75, 48.6195) -> (-20.25, 44.2894)
  line L370 (-20.25, 44.2894) -> (-25.25, 44.2894)
  line L371 (-25.25, 44.2894) -> (-27.75, 48.6195)
  line L372 (-16.75, 67.6721) -> (-14.25, 72.0022)
  line L373 (-14.25, 72.0022) -> (-9.25, 72.0022)
  line L374 (-9.25, 72.0022) -> (-6.75, 67.6721)
  line L375 (-6.75, 67.6721) -> (-9.25, 63.342)
  line L376 (-9.25, 63.342) -> (-14.25, 63.342)
  line L377 (-14.25, 63.342) -> (-16.75, 67.6721)
  line L378 (-33.25, 39.0933) -> (-30.75, 43.4234)
  line L379 (-30.75, 43.4234) -> (-25.75, 43.4234)
  line L380 (-25.75, 43.4234) -> (-23.25, 39.0933)
  line L381 (-23.25, 39.0933) -> (-25.75, 34.7631)
  line L382 (-25.75, 34.7631) -> (-30.75, 34.7631)
  line L383 (-30.75, 34.7631) -> (-33.25, 39.0933)
  line L384 (-11.25, 77.1984) -> (-8.75, 81.5285)
  line L385 (-8.75, 81.5285) -> (-3.75, 81.5285)
  line L386 (-3.75, 81.5285) -> (-1.25, 77.1984)
  line L387 (-1.25, 77.1984) -> (-3.75, 72.8683)
  line L388 (-3.75, 72.8683) -> (-8.75, 72.8683)
  line L389 (-8.75, 72.8683) -> (-11.25, 77.1984)
  line L390 (-38.75, 29.567) -> (-36.25, 33.8971)
  line L391 (-36.25, 33.8971) -> (-31.25, 33.8971)
  line L392 (-31.25, 33.8971) -> (-28.75, 29.567)
  line L393 (-28.75, 29.567) -> (-31.25, 25.2369)
  line L394 (-31.25, 25.2369) -> (-36.25, 25.2369)
  line L395 (-36.25, 25.2369) -> (-38.75, 29.567)
  line L396 (-5.75, 86.7247) -> (-3.25, 91.0548)
  line L397 (-3.25, 91.0548) -> (1.75, 91.0548)
  line L398 (1.75, 91.0548) -> (4.25, 86.7247)
  line L399 (4.25, 86.7247) -> (1.75, 82.3945)
  line L400 (1.75, 82.3945) -> (-3.25, 82.3945)
  line L401 (-3.25, 82.3945) -> (-5.75, 86.7247)
  line L402 (-44.25, 20.0407) -> (-41.75, 24.3708)
  line L403 (-41.75, 24.3708) -> (-36.75, 24.3708)
  line L404 (-36.75, 24.3708) -> (-34.25, 20.0407)
  line L405 (-34.25, 20.0407) -> (-36.75, 15.7106)
  line L406 (-36.75, 15.7106) -> (-41.75, 15.7106)
  line L407 (-41.75, 15.7106) -> (-44.25, 20.0407)
  line L408 (-0.25, 96.2509) -> (2.25, 100.5811)
  line L409 (2.25, 100.5811) -> (7.25, 100.5811)
  line L410 (7.25, 100.5811) -> (9.75, 96.2509)
  line L411 (9.75, 96.2509) -> (7.25, 91.9208)
  line L412 (7.25, 91.9208) -> (2.25, 91.9208)
  line L413 (2.25, 91.9208) -> (-0.25, 96.2509)
  line L414 (-49.75, 10.5144) -> (-47.25, 14.8446)
  line L415 (-47.25, 14.8446) -> (-42.25, 14.8446)
  line L416 (-42.25, 14.8446) -> (-39.75, 10.5144)
  line L417 (-39.75, 10.5144) -> (-42.25, 6.1843)
  line L418 (-42.25, 6.1843) -> (-47.25, 6.1843)
  line L419 (-47.25, 6.1843) -> (-49.75, 10.5144)
  line L420 (16.25, -8.5381) -> (18.75, -4.208)
  line L421 (18.75, -4.208) -> (23.75, -4.208)
  line L422 (23.75, -4.208) -> (26.25, -8.5381)
  line L423 (26.25, -8.5381) -> (23.75, -12.8683)
  line L424 (23.75, -12.8683) -> (18.75, -12.8683)
  line L425 (18.75, -12.8683) -> (16.25, -8.5381)
  line L426 (10.75, -18.0644) -> (13.25, -13.7343)
  line L427 (13.25, -13.7343) -> (18.25, -13.7343)
  line L428 (18.25, -13.7343) -> (20.75, -18.0644)
  line L429 (20.75, -18.0644) -> (18.25, -22.3945)
  line L430 (18.25, -22.3945) -> (13.25, -22.3945)
  line L431 (13.25, -22.3945) -> (10.75, -18.0644)
  line L432 (21.75, 0.9881) -> (24.25, 5.3183)
  line L433 (24.25, 5.3183) -> (29.25, 5.3183)
  line L434 (29.25, 5.3183) -> (31.75, 0.9881)
  line L435 (31.75, 0.9881) -> (29.25, -3.342)
  line L436 (29.25, -3.342) -> (24.25, -3.342)
  line L437 (24.25, -3.342) -> (21.75, 0.9881)
  line L438 (5.25, -27.5907) -> (7.75, -23.2606)
  line L439 (7.75, -23.2606) -> (12.75, -23.2606)
  line L440 (12.75, -23.2606) -> (15.25, -27.5907)
  line L441 (15.25, -27.5907) -> (12.75, -31.9208)
  line L442 (12.75, -31.9208) -> (7.75, -31.9208)
  line L443 (7.75, -31.9208) -> (5.25, -27.5907)
  line L444 (27.25, 10.5144) -> (29.75, 14.8446)
  line L445 (29.75, 14.8446) -> (34.75, 14.8446)
  line L446 (34.75, 14.8446) -> (37.25, 10.5144)
  line L447 (37.25, 10.5144) -> (34.75, 6.1843)
  line L448 (34.75, 6.1843) -> (29.75, 6.1843)
  line L449 (29.75, 6.1843) -> (27.25, 10.5144)
  line L450 (-0.25, -37.117) -> (2.25, -32.7868)
  line L451 (2.25, -32.7868) -> (7.25, -32.7868)
  line L452 (7.25, -32.7868) -> (9.75, -37.117)
  line L453 (9.75, -37.117) -> (7.25, -41.4471)
  line L454 (7.25, -41.4471) -> (2.25, -41.4471)
  line L455 (2.25, -41.4471) -> (-0.25, -37.117)
  line L456 (32.75, 20.0407) -> (35.25, 24.3708)
  line L457 (35.25, 24.3708) -> (40.25, 24.3708)
  line L458 (40.25, 24.3708) -> (42.75, 20.0407)
  line L459 (42.75, 20.0407) -> (40.25, 15.7106)
  line L460 (40.25, 15.7106) -> (35.25, 15.7106)
  line L461 (35.25, 15.7106) -> (32.75, 20.0407)
  line L462 (-5.75, -46.6432) -> (-3.25, -42.3131)
  line L463 (-3.25, -42.3131) -> (1.75, -42.3131)
  line L464 (1.75, -42.3131) -> (4.25, -46.6432)
  line L465 (4.25, -46.6432) -> (1.75, -50.9734)
  line L466 (1.75, -50.9734) -> (-3.25, -50.9734)
  line L467 (-3.25, -50.9734) -> (-5.75, -46.6432)
  line L468 (38.25, 29.567) -> (40.75, 33.8971)
  line L469 (40.75, 33.8971) -> (45.75, 33.8971)
  line L470 (45.75, 33.8971) -> (48.25, 29.567)
  line L471 (48.25, 29.567) -> (45.75, 25.2369)
  line L472 (45.75, 25.2369) -> (40.75, 25.2369)
  line L473 (40.75, 25.2369) -> (38.25, 29.567)
  line L474 (-11.25, -56.1695) -> (-8.75, -51.8394)
  line L475 (-8.75, -51.8394) -> (-3.75, -51.8394)
  line L476 (-3.75, -51.8394) -> (-1.25, -56.1695)
  line L477 (-1.25, -56.1695) -> (-3.75, -60.4997)
  line L478 (-3.75, -60.4997) -> (-8.75, -60.4997)
  line L479 (-8.75, -60.4997) -> (-11.25, -56.1695)
  line L480 (-27.75, 67.6721) -> (-25.25, 72.0022)
  line L481 (-25.25, 72.0022) -> (-20.25, 72.0022)
  line L482 (-20.25, 72.0022) -> (-17.75, 67.6721)
  line L483 (-17.75, 67.6721) -> (-20.25, 63.342)
  line L484 (-20.25, 63.342) -> (-25.25, 63.342)
  line L485 (-25.25, 63.342) -> (-27.75, 67.6721)
  line L486 (-33.25, 58.1458) -> (-30.75, 62.476)
  line L487 (-30.75, 62.476) -> (-25.75, 62.476)
  line L488 (-25.75, 62.476) -> (-23.25, 58.1458)
  line L489 (-23.25, 58.1458) -> (-25.75, 53.8157)
  line L490 (-25.75, 53.8157) -> (-30.75, 53.8157)
  line L491 (-30.75, 53.8157) -> (-33.25, 58.1458)
  line L492 (-22.25, 77.1984) -> (-19.75, 81.5285)
  line L493 (-19.75, 81.5285) -> (-14.75, 81.5285)
  line L494 (-14.75, 81.5285) -> (-12.25, 77.1984)
  line L495 (-12.25, 77.1984) -> (-14.75, 72.8683)
  line L496 (-14.75, 72.8683) -> (-19.75, 72.8683)
  line L497 (-19.75, 72.8683) -> (-22.25, 77.1984)
  line L498 (-38.75, 48.6195) -> (-36.25, 52.9497)
  line L499 (-36.25, 52.9497) -> (-31.25, 52.9497)
  line L500 (-31.25, 52.9497) -> (-28.75, 48.6195)
  line L501 (-28.75, 48.6195) -> (-31.25, 44.2894)
  line L502 (-31.25, 44.2894) -> (-36.25, 44.2894)
  line L503 (-36.25, 44.2894) -> (-38.75, 48.6195)
  line L504 (-16.75, 86.7247) -> (-14.25, 91.0548)
  line L505 (-14.25, 91.0548) -> (-9.25, 91.0548)
  line L506 (-9.25, 91.0548) -> (-6.75, 86.7247)
  line L507 (-6.75, 86.7247) -> (-9.25, 82.3945)
  line L508 (-9.25, 82.3945) -> (-14.25, 82.3945)
  line L509 (-14.25, 82.3945) -> (-16.75, 86.7247)
  line L510 (-44.25, 39.0933) -> (-41.75, 43.4234)
  line L511 (-41.75, 43.4234) -> (-36.75, 43.4234)
  line L512 (-36.75, 43.4234) -> (-34.25, 39.0933)
  line L513 (-34.25, 39.0933) -> (-36.75, 34.7631)
  line L514 (-36.75, 34.7631) -> (-41.75, 34.7631)
  line L515 (-41.75, 34.7631) -> (-44.25, 39.0933)
  line L516 (-11.25, 96.2509) -> (-8.75, 100.5811)
  line L517 (-8.75, 100.5811) -> (-3.75, 100.5811)
  line L518 (-3.75, 100.5811) -> (-1.25, 96.2509)
  line L519 (-1.25, 96.2509) -> (-3.75, 91.9208)
  line L520 (-3.75, 91.9208) -> (-8.75, 91.9208)
  line L521 (-8.75, 91.9208) -> (-11.25, 96.2509)
  line L522 (-49.75, 29.567) -> (-47.25, 33.8971)
  line L523 (-47.25, 33.8971) -> (-42.25, 33.8971)
  line L524 (-42.25, 33.8971) -> (-39.75, 29.567)
  line L525 (-39.75, 29.567) -> (-42.25, 25.2369)
  line L526 (-42.25, 25.2369) -> (-47.25, 25.2369)
  line L527 (-47.25, 25.2369) -> (-49.75, 29.567)
  line L528 (-5.75, 105.7772) -> (-3.25, 110.1073)
  line L529 (-3.25, 110.1073) -> (1.75, 110.1073)
  line L530 (1.75, 110.1073) -> (4.25, 105.7772)
  line L531 (4.25, 105.7772) -> (1.75, 101.4471)
  line L532 (1.75, 101.4471) -> (-3.25, 101.4471)
  line L533 (-3.25, 101.4471) -> (-5.75, 105.7772)
  line L534 (-55.25, 20.0407) -> (-52.75, 24.3708)
  line L535 (-52.75, 24.3708) -> (-47.75, 24.3708)
  line L536 (-47.75, 24.3708) -> (-45.25, 20.0407)
  line L537 (-45.25, 20.0407) -> (-47.75, 15.7106)
  line L538 (-47.75, 15.7106) -> (-52.75, 15.7106)
  line L539 (-52.75, 15.7106) -> (-55.25, 20.0407)
  line L540 (21.75, -18.0644) -> (24.25, -13.7343)
  line L541 (24.25, -13.7343) -> (29.25, -13.7343)
  line L542 (29.25, -13.7343) -> (31.75, -18.0644)
  line L543 (31.75, -18.0644) -> (29.25, -22.3945)
  line L544 (29.25, -22.3945) -> (24.25, -22.3945)
  line L545 (24.25, -22.3945) -> (21.75, -18.0644)
  line L546 (16.25, -27.5907) -> (18.75, -23.2606)
  line L547 (18.75, -23.2606) -> (23.75, -23.2606)
  line L548 (23.75, -23.2606) -> (26.25, -27.5907)
  line L549 (26.25, -27.5907) -> (23.75, -31.9208)
  line L550 (23.75, -31.9208) -> (18.75, -31.9208)
  line L551 (18.75, -31.9208) -> (16.25, -27.5907)
  line L552 (27.25, -8.5381) -> (29.75, -4.208)
  line L553 (29.75, -4.208) -> (34.75, -4.208)
  line L554 (34.75, -4.208) -> (37.25, -8.5381)
  line L555 (37.25, -8.5381) -> (34.75, -12.8683)
  line L556 (34.75, -12.8683) -> (29.75, -12.8683)
  line L557 (29.75, -12.8683) -> (27.25, -8.5381)
  line L558 (10.75, -37.117) -> (13.25, -32.7868)
  line L559 (13.25, -32.7868) -> (18.25, -32.7868)
  line L560 (18.25, -32.7868) -> (20.75, -37.117)
  line L561 (20.75, -37.117) -> (18.25, -41.4471)
  line L562 (18.25, -41.4471) -> (13.25, -41.4471)
  line L563 (13.25, -41.4471) -> (10.75, -37.117)
  line L564 (32.75, 0.9881) -> (35.25, 5.3183)
  line L565 (35.25, 5.3183) -> (40.25, 5.3183)
  line L566 (40.25, 5.3183) -> (42.75, 0.9881)
  line L567 (42.75, 0.9881) -> (40.25, -3.342)